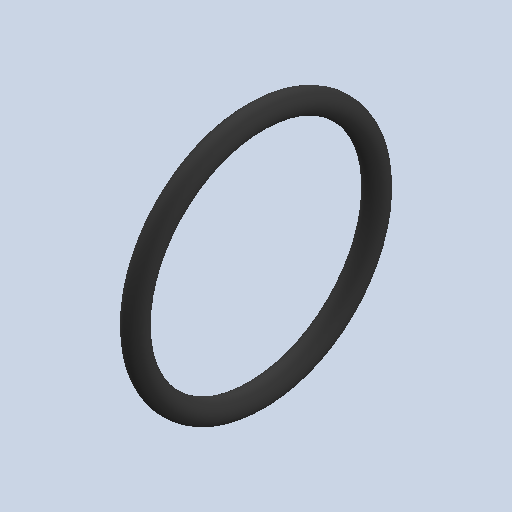
# Autodesk Inventor part: sealing_ring_V1
Saved by Autodesk Inventor 2023 (Build 270158000, 158)
## iProperties
Created: 2023-02-13
Part Number: sealing_ring_V1
Material: Gummi
Document SubType Name: Modeling
Designer: Mathi
Density: 0.93 g/cm^3
Appearance: Gummi - Schwarz
Author: Mathi
Autodesk Inventor part; units mm, degrees
ref_plane "YZ Plane" through (0, 0, 0) normal (1, 0, 0) x (0, 1, 0)
ref_plane "XZ Plane" through (0, 0, 0) normal (0, 1, 0) x (-1, 0, 0)
ref_plane "XY Plane" through (0, 0, 0) normal (0, 0, 1) x (1, 0, 0)
sketch "Skizze1" plane through (0, 0, 0) normal (0, 0, 1) x (1, 0, 0)
  line L0 (-14.8726, 0) -> (10.6884, 0)
  circle A0 centre (0, 27.5) radius 2.5
  line L1 (0, 0) -> (0, 27.5) construction
  dimension "d0" = 5
  dimension "d1" = 55
  constraints: 4 end point, 1 centre point, 1 horizontal, 1 point on line, 1 vertical
  measures "d0" diameter of A0
  measures "d1" diameter of L1.end L0
revolve "Umdrehung1" add sketch "Skizze1" angle 360 about axis through (-14.8726, 0, 0) along (1, 0, 0)
